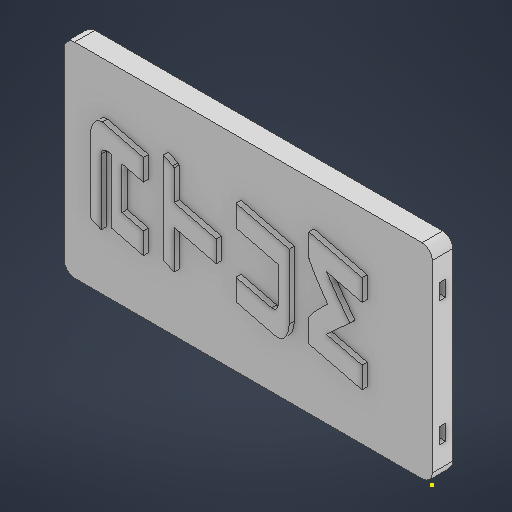
# Autodesk Inventor part: custom  plate vertical
Saved by Autodesk Inventor 2025.1 (Build 291241000, 241)
## iProperties
Created: 2024-12-05
Part Number: custom  plate vertical
Material: Generic
Document SubType Name: Modeling
Designer: Hunter Mathis
Density: 1 g/cm^3
Appearance: Default
Author: Hunter Mathis
Autodesk Inventor part; units mm, degrees
ref_plane "YZ Plane" through (0, 0, 0) normal (1, 0, 0) x (0, 1, 0)
ref_plane "XZ Plane" through (0, 0, 0) normal (0, 1, 0) x (-1, 0, 0)
ref_plane "XY Plane" through (0, 0, 0) normal (0, 0, 1) x (1, 0, 0)
sketch "Sketch1" plane through (0, 0, 0) normal (0, 0, 1) x (1, 0, 0)
  line L0 (0, 0) -> (-114.3, 0)
  line L1 (-114.3, 0) -> (-114.3, 63.5)
  line L2 (-114.3, 63.5) -> (0, 63.5)
  line L3 (0, 63.5) -> (0, 0)
  dimension "d7" = 114.3
  dimension "d8" = 63.5
  constraints: 8 end point, 2 parallel, 1 horizontal, 1 perpendicular
  measures "d7" distance of L1.end L2.end
  measures "d8" distance of L0.end L1.end
extrude "Extrusion1" add sketch "Sketch1" along normal blind 6.35
sketch "Sketch2" plane through (0, 0, 6.35) normal (0, 0, 1) x (1, 0, 0)
  line L0 (0, 0) -> (0, 63.5) projected
  line L1 (-114.3, 63.5) -> (-114.3, 0) projected
  line L2 (-114.3, 0) -> (0, 0) projected
  line L3 (0, 63.5) -> (-114.3, 63.5) projected
sketch "Sketch3" plane through (0, 0, 6.35) normal (0, 0, 1) x (1, 0, 0)
  line L0 (-110.6716, 35.2666) -> (-52.0005, 35.2666) construction
  line L1 (-52.0005, 35.2666) -> (-52.0005, 28.3217) construction
  line L2 (-52.0005, 28.3217) -> (-110.6716, 28.3217) construction
  line L3 (-110.6716, 28.3217) -> (-110.6716, 35.2666) construction
  line L4 (-114.3, 63.5) -> (-114.3, 0) projected
  point P0 (0, 0)
  constraints: 2 other
extrude "Extrusion2" [suppressed]
fillet "Fillet2" radius 3.175 4 edges at (-114.3, 63.5, 3.175) (-114.3, 0, 3.175) (0, 0, 3.175) (0, 63.5, 3.175)
sketch "Sketch4" plane through (0, 0, 6.35) normal (0, 0, 1) x (1, 0, 0)
  point P0 (0, 0)
sketch "Sketch5" plane through (0, 0, 6.35) normal (0, 0, 1) x (1, 0, 0)
  point P0 (0, 0)
sketch "Sketch6" plane through (0, 0, 6.35) normal (0, 0, 1) x (1, 0, 0)
  point P0 (0, 0)
ref_plane "Work Plane1" through (-57.15, 3.175, 0) normal (1, 0, 0) x (0, 0, -1)
sketch "Sketch7" plane through (-111.125, 63.5, 0) normal (0, 1, 0) x (1, 0, 0)
  line L0 (107.95, -6.35) -> (0, -6.35) projected
  line L1 (107.95, 0) -> (0, 0) projected
  line L2 (0, -6.35) -> (0, -3.175)
  line L3 (0, -6.35) -> (0, 0) projected
  line L4 (0, 0) -> (0, -6.35) projected
  line L5 (0, -6.35) -> (0, -3.5306)
  line L6 (0, -3.5306) -> (6.985, -3.5306)
  line L7 (6.985, -3.5306) -> (11.8618, -3.5306)
  line L8 (11.8618, -3.5306) -> (11.8618, -1.651)
  line L9 (11.8618, -1.651) -> (6.985, -1.651)
  line L10 (6.985, -1.651) -> (6.985, -3.5306)
  point P0 (111.125, 0)
  dimension "d24" = 4.8768
  dimension "d25" = 1.8796
  dimension "d26" = 2.8194
  dimension "d27" = 6.985
  constraints: 14 end point, 2 horizontal, 2 parallel, 1 midpoint, 1 perpendicular, 1 point on line
  measures "d24" distance of L6.end L7.end
  measures "d25" distance of L7.end L8.end
  measures "d26" distance between parallel lines of L6 L0
  measures "d27" distance of L5.end L6.end
extrude "Extrusion3" [suppressed]
sketch "Sketch8" plane through (-111.125, 0, 0) normal (0, -1, 0) x (1, 0, 0)
  line L0 (0, 0) -> (0, 6.35) projected
  line L1 (6.985, 3.5306) -> (6.985, 1.651) projected
  line L2 (11.8618, 1.651) -> (11.8618, 3.5306) projected
  line L3 (6.985, 1.651) -> (11.8618, 1.651)
  line L4 (11.8618, 1.651) -> (11.8618, 3.5306)
  line L5 (11.8618, 3.5306) -> (6.985, 3.5306)
  line L6 (6.985, 3.5306) -> (6.985, 1.651)
  line L7 (0, 0) -> (107.95, 0) projected
  point P0 (111.125, 0)
  constraints: 8 end point, 2 parallel, 1 horizontal, 1 perpendicular
extrude "Extrusion4" [suppressed]
mirror "Mirror1" [suppressed]
mirror "Mirror2" [suppressed]
sketch "Sketch9" plane through (0, 0, 6.35) normal (0, 0, 1) x (1, 0, 0)
  point P0 (0, 0)
sketch "Sketch10" plane through (0, 0, 6.35) normal (0, 0, 1) x (1, 0, 0)
  line L0 (-104.6693, 14.8634) -> (-104.6693, 18.0941) construction
  line L1 (-104.6693, 18.0941) -> (-86.5659, 18.0941) construction
  line L2 (-86.5659, 18.0941) -> (-86.5659, 14.8634) construction
  line L3 (-86.5659, 14.8634) -> (-104.6693, 14.8634) construction
  line L4 (-114.3, 60.325) -> (-114.3, 3.175) projected
  line L5 (-114.3, 60.325) -> (-114.3, 3.175)
  line L6 (-114.3, 3.175) -> (-114.3, 31.75)
  line L7 (0, 3.175) -> (0, 60.325) projected
  line L8 (-88.1593, 18.3152) -> (-98.2071, 20.8305)
  line L9 (-98.2071, 20.8305) -> (-98.2071, 40.5917)
  line L10 (-98.2071, 40.5917) -> (-99.1704, 40.8191)
  spline S0 degree 2 poles (-99.1704, 40.8191) (-99.5986, 40.9262) (-100.3612, 40.6987) (-100.9365, 40.1903) (-101.271, 39.4411) (-101.271, 39.0397) knots 0 0 0 1 2 3 4 4 4
  line L11 (-101.271, 39.0397) -> (-101.271, 18.7166)
  spline S1 degree 2 poles (-101.271, 18.7166) (-101.9533, 19.0243) (-103.5722, 19.7602) (-104.2545, 20.1214) knots 0 0 0 1 2 2 2
  line L12 (-104.2545, 20.1214) -> (-104.6693, 20.4425)
  line L13 (-104.6693, 20.4425) -> (-104.6693, 42.5049)
  spline S2 degree 2 poles (-104.6693, 42.5049) (-104.6693, 43.3612) (-104.201, 45.2744) (-103.2511, 46.8933) (-101.873, 47.9369) (-100.9231, 47.9101) knots 0 0 0 1 2 3 4 4 4
  line L14 (-100.9231, 47.9101) -> (-88.1593, 44.7259)
  line L15 (-88.1593, 44.7259) -> (-88.1593, 38.0764)
  line L16 (-88.1593, 38.0764) -> (-94.8088, 39.722)
  line L17 (-94.8088, 39.722) -> (-94.8088, 26.6104)
  line L18 (-94.8088, 26.6104) -> (-88.1593, 24.9647)
  line L19 (-88.1593, 24.9647) -> (-88.1593, 18.3152)
  spline S3 degree 2 poles (-78.6284, 18.6898) (-79.3107, 18.9976) (-80.9296, 19.7334) (-81.612, 20.0947) knots 0 0 0 1 2 2 2
  line L20 (-81.612, 20.0947) -> (-82.0267, 20.4158)
  line L21 (-82.0267, 20.4158) -> (-82.0267, 48.4453)
  spline S4 degree 2 poles (-82.0267, 48.4453) (-81.3444, 48.1777) (-79.7255, 47.4151) (-79.0432, 47.0271) knots 0 0 0 1 2 2 2
  line L22 (-79.0432, 47.0271) -> (-78.6284, 46.706)
  line L23 (-78.6284, 46.706) -> (-78.6284, 37.3673)
  line L24 (-78.6284, 37.3673) -> (-65.5167, 34.1027)
  line L25 (-65.5167, 34.1027) -> (-65.5167, 27.4532)
  line L26 (-65.5167, 27.4532) -> (-78.6284, 30.7178)
  line L27 (-78.6284, 30.7178) -> (-78.6284, 18.6898)
  spline S5 degree 2 poles (-46.6203, 17.1111) (-45.6704, 17.0843) (-44.2923, 18.1145) (-43.3424, 19.7334) (-42.8741, 21.6466) (-42.8741, 22.5029) knots 0 0 0 1 2 3 4 4 4
  line L28 (-42.8741, 22.5029) -> (-42.8741, 42.7056)
  line L29 (-42.8741, 42.7056) -> (-59.3841, 46.813)
  line L30 (-59.3841, 46.813) -> (-59.3841, 40.1635)
  line L31 (-59.3841, 40.1635) -> (-46.2725, 36.899)
  line L32 (-46.2725, 36.899) -> (-46.2725, 25.9548)
  spline S6 degree 2 poles (-46.2725, 25.9548) (-46.2725, 25.5668) (-46.607, 24.8309) (-47.1823, 24.3091) (-47.9449, 24.0817) (-48.3596, 24.1753) knots 0 0 0 1 2 3 4 4 4
  line L33 (-48.3596, 24.1753) -> (-59.3841, 26.9315)
  line L34 (-59.3841, 26.9315) -> (-59.3841, 20.282)
  line L35 (-59.3841, 20.282) -> (-46.6203, 17.1111)
  line L36 (-36.7416, 20.282) -> (-20.2316, 16.1745)
  line L37 (-20.2316, 16.1745) -> (-20.2316, 22.824)
  line L38 (-20.2316, 22.824) -> (-31.2695, 25.5668)
  spline S7 degree 2 poles (-31.2695, 25.5668) (-30.5871, 26.3026) (-28.8879, 27.9215) (-27.0015, 29.6207) (-25.0213, 31.3199) (-24.0447, 32.1627) knots 0 0 0 1 2 3 4 4 4
  line L39 (-24.0447, 32.1627) -> (-24.0447, 32.243)
  spline S8 degree 2 poles (-24.0447, 32.243) (-25.0213, 33.5542) (-27.0282, 36.2702) (-28.9147, 38.8925) (-30.5871, 41.3677) (-31.2695, 42.4514) knots 0 0 0 1 2 3 4 4 4
  line L40 (-31.2695, 42.4514) -> (-20.2316, 39.6953)
  line L41 (-20.2316, 39.6953) -> (-20.2316, 46.3448)
  line L42 (-20.2316, 46.3448) -> (-36.7416, 50.4522)
  line L43 (-36.7416, 50.4522) -> (-36.7416, 43.2541)
  spline S9 degree 2 poles (-36.7416, 43.2541) (-36.3536, 42.4246) (-35.2699, 40.4846) (-33.9721, 38.4109) (-32.5271, 36.2702) (-31.7912, 35.1731) knots 0 0 0 1 2 3 4 4 4
  line L44 (-31.7912, 35.1731) -> (-30.9617, 33.9154)
  spline S10 degree 2 poles (-30.9617, 33.9154) (-33.0757, 31.8416) (-35.979, 28.8179) (-36.7416, 27.48) knots 0 0 0 1 2 2 2
  line L45 (-36.7416, 27.48) -> (-36.7416, 20.282)
  point P0 (0, 0)
  constraints: 4 end point, 1 collinear, 1 midpoint, 2 other
sketch "Sketch11" plane through (0, 3.175, 0) normal (1, 0, 0) x (0, 0, -1)
  line L0 (0, 0) -> (-6.35, 0) projected
  line L1 (-3.175, 0) -> (-3.175, 8.89)
  line L2 (-4.1148, 6.4516) -> (-2.2352, 6.4516)
  line L3 (-2.2352, 6.4516) -> (-2.2352, 11.3284)
  line L4 (-2.2352, 11.3284) -> (-4.1148, 11.3284)
  line L5 (-4.1148, 11.3284) -> (-4.1148, 6.4516)
  line L6 (-4.1148, 6.4516) -> (-2.2352, 11.3284) construction
  line L7 (-2.2352, 6.4516) -> (-4.1148, 11.3284) construction
  line L8 (0, 60.325) -> (-6.35, 60.325) projected
  line L9 (-3.175, 60.325) -> (-3.175, 47.625)
  line L10 (-4.1148, 45.1866) -> (-2.2352, 45.1866)
  line L11 (-2.2352, 45.1866) -> (-2.2352, 50.0634)
  line L12 (-2.2352, 50.0634) -> (-4.1148, 50.0634)
  line L13 (-4.1148, 50.0634) -> (-4.1148, 45.1866)
  line L14 (-4.1148, 45.1866) -> (-2.2352, 50.0634) construction
  line L15 (-2.2352, 45.1866) -> (-4.1148, 50.0634) construction
  point P0 (0, -3.175)
  point P1 (-2.2352, 47.625)
  dimension "d29" = 8.89
  dimension "d30" = 12.7
  dimension "d31" = 4.8768
  dimension "d32" = 1.8796
  dimension "d33" = 4.8768
  dimension "d34" = 1.8796
  constraints: 28 end point, 7 midpoint, 4 parallel, 2 horizontal, 2 perpendicular, 2 vertical
  measures "d29" distance of L1.start L1.end
  measures "d30" distance of L9.start L9.end
  measures "d31" distance between parallel lines of L12 L10
  measures "d32" distance from line of point (-2.235, 47.625) L13
  measures "d33" distance between parallel lines of L4 L2
  measures "d34" distance between parallel lines of L3 L5
extrude "Extrusion5" cut sketch "Sketch11" against normal blind 9.652
extrude "Extrusion6" add sketch "Sketch10" along normal blind 1.5875
body "Solid1"
